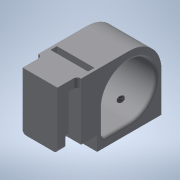
# Autodesk Inventor part: LoopD
Saved by Autodesk Inventor 2022 (Build 260153000, 153)
## iProperties
Created: 2014-06-16
Part Number: LoopD
Material: Generisch
Document SubType Name: Modeling
Designer: g.schardt
Density: 1 g/cm^3
Appearance: Vorgabe
Author: g.schardt
Autodesk Inventor part; units mm, degrees
ref_plane "YZ Plane" through (0, 0, 0) normal (1, 0, 0) x (0, 1, 0)
ref_plane "XZ Plane" through (0, 0, 0) normal (0, 1, 0) x (-1, 0, 0)
ref_plane "XY Plane" through (0, 0, 0) normal (0, 0, 1) x (1, 0, 0)
sketch "Skizze1" plane through (0, 0, 0) normal (1, 0, 0) x (0, 1, 0)
  line L0 (-24, -16.9753) -> (-15, -16.9753)
  line L1 (21, -18) -> (21, 15.0247)
  line L2 (21, 15.0247) -> (-24, 15.0247)
  line L3 (-24, 15.0247) -> (-24, -16.9753)
  line L4 (-15, -16.9753) -> (-15, -24.9753)
  line L5 (-15, -24.9753) -> (21, -24.9753)
  line L6 (21, -24.9753) -> (21, -18)
  point P0 (0, 0)
  dimension "d43" = 36
  dimension "d45" = 40
  dimension "d46" = 45
  dimension "d47" = 32
  constraints: 14 end point, 4 parallel, 1 horizontal, 1 perpendicular
  measures "d43" distance of L5.end L4.end
  measures "d45" distance between parallel lines of L5 L2
  measures "d46" distance of L1.end L2.end
  measures "d47" distance of L2.end L0.start
extrude "Extrusion1" add sketch "Skizze1" along normal blind 24
sketch "Skizze2" plane through (24, 0, 0) normal (1, 0, 0) x (0, 0, -1)
  line L0 (24.9753, 21) -> (-15.0247, 21) projected
  line L1 (-10.0247, 18) -> (19.9753, 18)
  line L2 (19.9753, 18) -> (19.9753, -12)
  line L3 (19.9753, -12) -> (-10.0247, -12)
  line L4 (-10.0247, -12) -> (-10.0247, 18)
  line L5 (24.9753, -15) -> (24.9753, 21) projected
  point P0 (18, 21)
  point P1 (0, 0)
  dimension "d4" = 30
  dimension "d5" = 30
  dimension "d6" = 3
  dimension "d49" = 5
  constraints: 8 end point, 2 parallel, 1 horizontal, 1 perpendicular
  measures "d4" distance of L1.start L1.end
  measures "d5" distance between parallel lines of L3 L1
  measures "d6" distance between parallel lines of L0 L1
  measures "d49" distance between parallel lines of L5 L2
extrude "Extrusion2" cut sketch "Skizze2" against normal through all
fillet "Rundung1" radius 15 1 edges at (12, 18, -19.9753)
fillet "Rundung2" radius 15 1 edges at (12, 18, 10.0247)
fillet "Rundung3" radius 18 1 edges at (12, 21, 15.0247)
sketch "Skizze5" plane through (0, -24, -16.9753) normal (0, 0, -1) x (-1, 0, 0)
  line L0 (-1.5, 9) -> (-22.5, 9)
  line L1 (-22.5, 9) -> (-22.5, 5.4)
  line L2 (-22.5, 5.4) -> (-1.5, 5.4)
  line L3 (-1.5, 5.4) -> (-1.5, 9)
  line L4 (0, 9) -> (-24, 9) projected
  line L5 (0, 9) -> (-24, 9) projected
  point P0 (0, 24)
  point P1 (-12, 5.4)
  point P2 (-12, 9)
  point P3 (-1.5, 9)
  point P4 (-22.5, 9)
  dimension "d50" = 21
  dimension "d51" = 3.6
  constraints: 8 end point, 2 midpoint, 2 parallel, 1 collinear, 1 horizontal, 1 perpendicular, 1 vertical alignment
  measures "d50" distance of L2.end L1.end
  measures "d51" distance of L1.end L0.end
extrude "Extrusion4" cut sketch "Skizze5" against normal through all
sketch "Skizze6" plane through (0, -15, -24.9753) normal (0, 0, -1) x (-1, 0, 0)
  line L0 (0, 36) -> (-24, 36) projected
  point P0 (0, 15)
  point P1 (-12, 25.2)
  point P2 (-12, 36)
  dimension "d55" = 10.8
  constraints: 1 midpoint, 1 vertical alignment
  measures "d55" distance from line of L0 point (-12, 25.2)
hole "Bohrung2" at (12, 10.2, -24.9753) direction (0, 0, 1) diameter 3.242 depth 11.8 tip angle 118 thread size "M4x0.7" class "6H" standard "ANSI Metric M Profile"
fillet "Rundung10" radius 15 1 edges at (12, -12, 10.0247)
fillet "Rundung12" radius 1.5 7 edges at (24, -12, -12.4753) (24, -4.5, -19.9753) (24, 13.6066, -15.5819) (0, -4.5, -19.9753) (0, -12, -12.4753) (0, 13.6066, -15.5819) (12, -12, -19.9753)
chamfer "Fase1" distance 0.5 angle 45 3 edges at (1.5, -16.8, -16.9753) (12, -18.6, -16.9753) (22.5, -16.8, -16.9753)
sketch "Skizze7" plane through (0, -24, -16.9753) normal (0, -1, 0) x (1, 0, 0)
  line L0 (2.25, 32) -> (21.75, 32)
  line L1 (21.75, 32) -> (21.75, 27)
  line L2 (21.75, 27) -> (2.25, 27)
  line L3 (2.25, 27) -> (2.25, 32)
  line L4 (0, 32) -> (24, 32) projected
  line L5 (7, 27) -> (17, 27)
  line L6 (17, 27) -> (17, 0)
  line L7 (17, 0) -> (7, 0)
  line L8 (7, 0) -> (7, 27)
  line L9 (0, 0) -> (24, 0) projected
  point P0 (12, 32)
  point P1 (12, 32)
  point P2 (12, 27)
  point P3 (12, 27)
  dimension "d73" = 19.5
  dimension "d74" = 5
  dimension "d75" = 10
  constraints: 16 end point, 4 midpoint, 4 parallel, 3 collinear, 2 coincident, 2 horizontal, 2 perpendicular
  measures "d73" distance of L1.end L2.end
  measures "d74" distance of L0.end L1.end
  measures "d75" distance of L5.start L5.end
extrude "Extrusion5" add sketch "Skizze7" along normal blind 6.5
sketch "Skizze8" plane through (0, -30.5, -16.9753) normal (0, -1, 0) x (1, 0, 0)
  line L0 (2.25, 32) -> (2.25, 27) projected
  line L1 (21.75, 27) -> (21.75, 32) projected
  line L2 (7, 0) -> (17, 0) projected
  line L3 (17, 0) -> (24, 0) projected
  line L4 (2.25, 32) -> (21.75, 32)
  line L5 (21.75, 32) -> (21.75, 0)
  line L6 (21.75, 0) -> (2.25, 0)
  line L7 (2.25, 0) -> (2.25, 32)
  constraints: 8 end point, 2 parallel, 1 horizontal, 1 perpendicular, 1 point on line
extrude "Extrusion6" add sketch "Skizze8" along normal blind 4.5
fillet "Rundung16" radius 2 6 edges at (21.75, -24, 12.5247) (21.75, -32.75, -16.9753) (17, -27.25, -16.9753) (2.25, -32.75, -16.9753) (7, -27.25, -16.9753) (2.25, -24, 12.5247)
